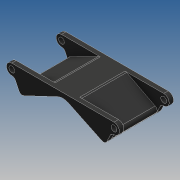
# Autodesk Inventor part: Front guard v2
Saved by Autodesk Inventor 2017 (Build 210142000, 142)
## iProperties
Created: 2017-07-08
Part Number: Front guard v2
Material: Generic
Document SubType Name: Modeling
Designer: yella
Density: 1 g/cm^3
Appearance: Rubber - Black
Author: yella
Autodesk Inventor part; units mm, degrees
ref_plane "YZ Plane" through (0, 0, 0) normal (1, 0, 0) x (0, 1, 0)
ref_plane "XZ Plane" through (0, 0, 0) normal (0, 1, 0) x (-1, 0, 0)
ref_plane "XY Plane" through (0, 0, 0) normal (0, 0, 1) x (1, 0, 0)
sketch "Sketch1" plane through (0, 0, 0) normal (0, 1, 0) x (-1, 0, 0)
  circle A0 centre (24, -57.282) radius 1.6
  circle A1 centre (-24, -57.282) radius 1.6
  circle A2 centre (30.6147, -73.9084) radius 1.6
  circle A3 centre (-30.6218, -73.9117) radius 1.6
  circle A4 centre (28.2679, -64.7437) radius 1.6
  circle A5 centre (-28.2698, -64.7437) radius 1.6
  line L0 (48.2265, -83.602) -> (45.2265, -83.602)
  line L1 (45.2265, -83.602) -> (45.2265, -77.602)
  line L2 (45.2265, -77.602) -> (48.2265, -77.602)
  line L3 (48.2265, -77.602) -> (48.2265, -83.602)
  line L4 (-45.2265, -83.602) -> (-48.2265, -83.602)
  line L5 (-48.2265, -83.602) -> (-48.2265, -77.602)
  line L6 (-48.2265, -77.602) -> (-45.2265, -77.602)
  line L7 (-45.2265, -77.602) -> (-45.2265, -83.602)
  line L8 (48.3297, -88.9448) -> (2.1402, -66.9582)
  line L9 (-2.1585, -66.9585) -> (-48.3297, -88.9448)
  arc A6 (2.1402, -66.9582) -> (-2.1585, -66.9585) centre (-0.0088, -71.4728) ccw
  line L10 (30.6147, -73.9084) -> (28.0518, -79.2924)
  line L11 (28.0518, -79.2924) -> (-28.0596, -79.2924)
  line L12 (-30.6218, -73.9117) -> (-28.0596, -79.2924)
  line L13 (-28.0596, -79.2924) -> (-28.9194, -77.4867)
  line L14 (28.0518, -79.2924) -> (28.9114, -77.4867)
  line L15 (2.9996, -65.1524) -> (21.6357, -74.0234)
  line L16 (-3.0185, -65.1529) -> (-21.6377, -74.0192)
  arc A7 (2.9996, -65.1524) -> (-3.0185, -65.1529) centre (-0.009, -71.4729) ccw
  line L17 (26.297, -68.8841) -> (23.4415, -74.883)
  line L18 (24.3011, -73.0771) -> (25.5905, -70.3683)
  line L19 (7.0641, -61.5496) -> (5.1533, -60.64)
  line L20 (-26.2983, -68.8839) -> (-24.3033, -73.0733)
  line L21 (-23.4434, -74.879) -> (-25.5914, -70.3683)
  line L22 (-5.1635, -60.6408) -> (-7.0717, -61.5494)
  arc A8 (5.1533, -60.64) -> (-5.1635, -60.6408) centre (-0.0043, -71.4751) ccw
  arc A9 (28.2679, -67.7437) -> (28.2679, -61.7437) centre (28.2679, -64.7437) ccw
  line L23 (28.2679, -64.7437) -> (28.2679, -61.7437) construction
  line L24 (28.2679, -64.7437) -> (31.2679, -64.7437) construction
  line L25 (28.2679, -64.7437) -> (28.2679, -67.7437) construction
  line L26 (28.2679, -61.7437) -> (7.9237, -61.7437)
  line L27 (28.2679, -67.7437) -> (28.1029, -67.7437)
  arc A10 (-28.2698, -61.7437) -> (-28.2698, -67.7437) centre (-28.2698, -64.7437) ccw
  line L28 (-28.2698, -64.7437) -> (-28.2698, -61.7437) construction
  line L29 (-28.2698, -64.7437) -> (-25.2698, -64.7437) construction
  line L30 (-28.2698, -67.7437) -> (-28.104, -67.7437)
  line L31 (-28.2698, -61.7437) -> (-7.9316, -61.7437)
  arc A11 (21.6357, -74.0234) -> (24.3011, -73.0771) centre (22.4953, -72.2175) ccw
  arc A12 (-24.3033, -73.0733) -> (-21.6377, -74.0192) centre (-22.4976, -72.2134) ccw
  arc A13 (-7.9316, -61.7437) -> (-7.0717, -61.5494) centre (-7.9316, -59.7437) ccw
  arc A14 (7.0641, -61.5496) -> (7.9237, -61.7437) centre (7.9237, -59.7437) ccw
  arc A15 (28.1029, -67.7437) -> (26.297, -68.8841) centre (28.1029, -69.7437) ccw
  arc A16 (-26.2983, -68.8839) -> (-28.104, -67.7437) centre (-28.104, -69.7437) ccw
  line L32 (28.2679, -61.7437) -> (-28.2698, -61.7437)
  point P0 (0, 0)
  dimension "d0" = 3.2
  dimension "d1" = 6
  dimension "d2" = 6
  dimension "d3" = 5
  dimension "d4" = 2
  dimension "d5" = 7
  dimension "d6" = 5
  dimension "d7" = 12
  dimension "d8" = 3
  dimension "d9" = 90
  dimension "d10" = 180
  dimension "d11" = 3
  dimension "d12" = 90
  dimension "d13" = 2
  dimension "d14" = 2
  constraints: 66 end point, 22 point on circle, 18 tangent, 17 centre point, 16 point on line, 11 perpendicular, 6 parallel, 5 horizontal, 4 coincident, 4 equal radius, 1 collinear
  measures "d0" diameter of A5
  measures "d1" distance of L1.start L2.start
  measures "d2" distance of L4.end L6.start
  measures "d3" radius of A6
  measures "d4" distance of L11.end L13.end
  measures "d5" radius of A7
  measures "d6" distance of L17.end L18.end
  measures "d7" radius of A8
  measures "d8" radius of A9
  measures "d9" angle of L24 L23
  measures "d10" angle of L23 L25
  measures "d11" radius of A10
  measures "d12" angle of L29 L28
  measures "d13" radius of A11
  measures "d14" radius of A15
extrude "Extrusion1" add sketch "Sketch1" along normal blind 2.5 contours A7 L16 A12 L20 A16 L30 A10 L31 L32 L26 A9 L27 A15 L17 A11 L15
sketch "Sketch2" plane through (0, 2.5, 0) normal (0, 1, 0) x (1, 0, 0)
  line L0 (-24.3011, 73.0771) -> (-26.297, 68.8841) projected
  line L1 (26.2983, 68.8839) -> (24.3033, 73.0733) projected
  arc A0 (-21.6357, 74.0234) -> (-24.3011, 73.0771) centre (-22.4953, 72.2175) ccw projected
  line L2 (-24.4649, 72.7332) -> (-24.3011, 73.0771)
  arc A1 (-24.4649, 72.7332) -> (-23.5723, 70.0943) centre (-22.659, 71.8736) ccw
  line L3 (24.4662, 72.7312) -> (24.3033, 73.0733)
  arc A2 (23.5739, 70.0921) -> (24.4662, 72.7312) centre (22.6605, 71.8713) ccw
  arc A3 (24.3033, 73.0733) -> (21.6377, 74.0192) centre (22.4976, 72.2134) ccw projected
  line L4 (21.6377, 74.0192) -> (3.0185, 65.1529) projected
  line L5 (-2.9996, 65.1524) -> (-21.6357, 74.0234) projected
  arc A4 (-2.9996, 65.1524) -> (3.0185, 65.1529) centre (0.009, 71.4729) ccw projected
  line L6 (-28.2679, 61.7437) -> (28.2698, 61.7437) projected
  line L7 (7.742, 61.9645) -> (23.5739, 70.0921)
  line L8 (-7.7335, 61.9644) -> (-23.5723, 70.0943)
  line L9 (-6.8202, 61.7437) -> (6.8286, 61.7437)
  arc A5 (6.8286, 61.7437) -> (7.742, 61.9645) centre (6.8286, 63.7437) ccw
  arc A6 (-7.7335, 61.9644) -> (-6.8202, 61.7437) centre (-6.8202, 63.7437) ccw
  point P0 (0, 0)
  point P1 (-5.1533, 60.64)
  point P2 (-25.2991, 70.9806)
  point P3 (25.3008, 70.9786)
  point P4 (7.312, 61.7437)
  point P5 (-7.3035, 61.7437)
  dimension "d17" = 2
  dimension "d18" = 2
  dimension "d23" = 2
  constraints: 10 end point, 8 point on circle, 8 point on line, 7 tangent, 4 centre point, 2 midpoint, 1 collinear, 1 equal radius
  measures "d17" radius of A1
  measures "d18" radius of A2
  measures "d23" radius of A5
extrude "Extrusion2" add sketch "Sketch2" along normal blind 25
sketch "Sketch3" plane through (0, 27.5, 0) normal (0, 1, 0) x (1, 0, 0)
  arc A0 (23.5739, 70.0921) -> (24.4662, 72.7312) centre (22.6605, 71.8713) ccw projected
  arc A1 (28.2698, 61.7437) -> (28.2698, 67.7437) centre (28.2698, 64.7437) ccw projected
  line L0 (28.2698, 67.7437) -> (28.104, 67.7437) projected
  arc A2 (26.2983, 68.8839) -> (28.104, 67.7437) centre (28.104, 69.7437) ccw projected
  line L1 (26.2983, 68.8839) -> (24.4662, 72.7312) projected
  circle A3 centre (28.2698, 64.7437) radius 1.6 projected
  arc A4 (23.5739, 70.0921) -> (24.4662, 72.7312) centre (22.6605, 71.8713) ccw projected
  line L2 (24.4662, 72.7312) -> (24.3033, 73.0733) projected
  arc A5 (24.3033, 73.0733) -> (21.6377, 74.0192) centre (22.4976, 72.2134) ccw projected
  line L3 (21.6377, 74.0192) -> (3.0185, 65.1529) projected
  arc A6 (-2.9996, 65.1524) -> (3.0185, 65.1529) centre (0.009, 71.4729) ccw projected
  line L4 (-2.9996, 65.1524) -> (-21.6357, 74.0234) projected
  arc A7 (-21.6357, 74.0234) -> (-24.3011, 73.0771) centre (-22.4953, 72.2175) ccw projected
  line L5 (-24.3011, 73.0771) -> (-24.4649, 72.7332) projected
  arc A8 (-24.4649, 72.7332) -> (-23.5723, 70.0943) centre (-22.659, 71.8736) ccw projected
  arc A9 (-24.4649, 72.7332) -> (-23.5723, 70.0943) centre (-22.659, 71.8736) ccw projected
  line L6 (-24.4649, 72.7332) -> (-26.297, 68.8841) projected
  arc A10 (-28.1029, 67.7437) -> (-26.297, 68.8841) centre (-28.1029, 69.7437) ccw projected
  line L7 (-28.1029, 67.7437) -> (-28.2679, 67.7437) projected
  arc A11 (-28.2679, 67.7437) -> (-28.2679, 61.7437) centre (-28.2679, 64.7437) ccw projected
  circle A12 centre (-28.2679, 64.7437) radius 1.6 projected
  arc A13 (-7.7335, 61.9644) -> (-6.8202, 61.7437) centre (-6.8202, 63.7437) ccw projected
  line L8 (-7.7335, 61.9644) -> (-23.5723, 70.0943) projected
  line L9 (-28.2679, 61.7437) -> (-6.8202, 61.7437) projected
  line L10 (-23.5723, 70.0943) -> (-7.7335, 61.9644) projected
  arc A14 (-7.7335, 61.9644) -> (-6.8202, 61.7437) centre (-6.8202, 63.7437) ccw projected
  line L11 (-6.8202, 61.7437) -> (6.8286, 61.7437) projected
  arc A15 (6.8286, 61.7437) -> (7.742, 61.9645) centre (6.8286, 63.7437) ccw projected
  line L12 (7.742, 61.9645) -> (23.5739, 70.0921) projected
  arc A16 (6.8286, 61.7437) -> (7.742, 61.9645) centre (6.8286, 63.7437) ccw projected
  line L13 (6.8286, 61.7437) -> (28.2698, 61.7437) projected
  line L14 (23.5739, 70.0921) -> (7.742, 61.9645) projected
  point P0 (0, 0)
extrude "Extrusion3" add sketch "Sketch3" along normal blind 2.5
body "Solid1"
